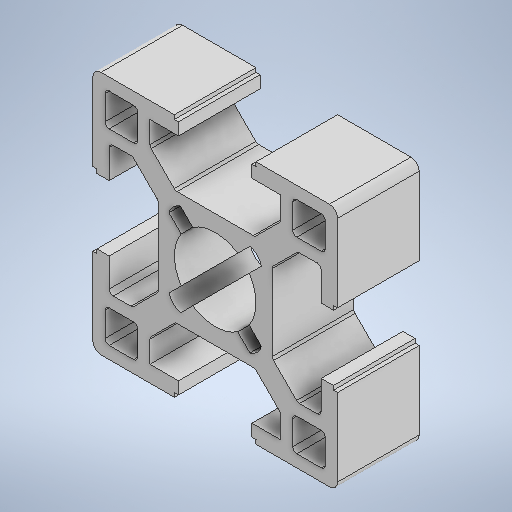
# Autodesk Inventor part: perfil_30x30_001
Saved by Autodesk Inventor 2026 (Build 300175000, 175)
## iProperties
Created: 2025-04-10
Part Number: perfil_30x30_001
Material: Generic
Document SubType Name: Modeling
Designer: Tony Dias
Density: 1 g/cm^3
Appearance: Default
Author: Tony Dias
Autodesk Inventor part; units mm, degrees
ref_plane "YZ Plane" through (0, 0, 0) normal (1, 0, 0) x (0, 1, 0)
ref_plane "XZ Plane" through (0, 0, 0) normal (0, 1, 0) x (-1, 0, 0)
ref_plane "XY Plane" through (0, 0, 0) normal (0, 0, 1) x (1, 0, 0)
sketch "Sketch1" plane through (0, 0, 0) normal (0, 0, 1) x (1, 0, 0)
  circle A0 centre (0, 0) radius 5 construction
  line L0 (-15, 15) -> (-4.5, 15) construction
  line L1 (-7, 7) -> (-7, 0) construction
  line L2 (-15, 15) -> (0, 0) construction
  line L3 (-7, 7) -> (0, 7) construction
  line L4 (-15, 15) -> (-15, 4) construction
  line L5 (-15, 4) -> (-13, 4) construction
  line L6 (-13.5, 13.5) -> (-9.5, 13.5)
  line L7 (-9.5, 13.5) -> (-9.5, 9.5)
  line L8 (-9.5, 9.5) -> (-13.5, 9.5)
  line L9 (-13.5, 9.5) -> (-13.5, 13.5)
  line L10 (-13.5, 13.5) -> (-9.5, 9.5) construction
  line L11 (-9.5, 13.5) -> (-13.5, 9.5) construction
  line L12 (-10.1213, 8) -> (-7, 4.8787)
  line L13 (-13, 8) -> (-10.1213, 8)
  line L14 (-13, 8) -> (-13, 4)
  line L15 (-7, 4.8787) -> (-7, 0)
  line L16 (-7, 0) -> (-5, 0)
  line L17 (-5.6712, 4.257) -> (-4.1712, 2.757)
  line L18 (-4.257, 5.6712) -> (-2.757, 4.1712)
  arc A1 (-4.257, 5.6712) -> (-5.6712, 4.257) centre (-3.7394, 3.7394) ccw
  arc A2 (0, 5) -> (-2.757, 4.1712) centre (0, 0) ccw
  arc A3 (-4.1712, 2.757) -> (-5, 0) centre (0, 0) ccw
  line L19 (-15, 4) -> (-14.5, 4) construction
  line L20 (-14.5, 4) -> (-14.5, 4.5)
  line L21 (-14.5, 4.5) -> (-15, 4.5)
  line L22 (-15, 4.5) -> (-15, 4) construction
  line L23 (-14.5, 4) -> (-13, 4)
  line L24 (-15, 15) -> (-15, 4.5)
  line L25 (-4.5, 15) -> (-4.5, 13) construction
  line L26 (-4.5, 13) -> (-8, 13)
  line L27 (-8, 13) -> (-8, 10.1213)
  line L28 (-8, 10.1213) -> (-4.8787, 7)
  line L29 (-4.8787, 7) -> (0, 7)
  line L30 (-4.5, 15) -> (-5, 15) construction
  line L31 (-5, 15) -> (-5, 14.5)
  line L32 (-5, 14.5) -> (-4.5, 14.5)
  line L33 (-4.5, 14.5) -> (-4.5, 15) construction
  line L34 (-4.5, 14.5) -> (-4.5, 13)
  line L35 (-15, 15) -> (-5, 15)
  line L36 (0, 7) -> (0, 5)
  point P0 (-11.5, 11.5)
  point P1 (-4.9212, 3.507)
  point P2 (-9.5, 11.5)
  dimension "d1" = 15
  dimension "d2" = 15
  dimension "d3" = 8
  dimension "d4" = 2
  dimension "d5" = 4
  dimension "d6" = 2
  dimension "d7" = 4
  dimension "d8" = 11.5
  dimension "d9" = 1.5
  dimension "d10" = 1.5
  dimension "d12" = 1.5
  dimension "d13" = 1
  dimension "d14" = 2
  dimension "d15" = 0.5
  dimension "d16" = 1.5
  constraints: 74 end point, 9 parallel, 9 point on circle, 8 equal length, 8 horizontal, 6 vertical, 5 collinear, 5 perpendicular, 4 centre point, 4 midpoint, 4 point on line, 3 concentric, 2 coincident, 2 vertical alignment, 1 horizontal alignment, 1 other
  measures "d1" horizontal distance of point (0, 0) L0.start
  measures "d2" horizontal distance of L0.start point (0, 0)
  measures "d3" distance from line of L0.start L1
  measures "d4" distance edge to line of A0 L1
  measures "d5" vertical distance of point (0, 0) L4.end
  measures "d6" distance of L4.end L5.end
  measures "d7" distance of L6.end L7.end
  measures "d8" horizontal distance of point (0, 0) point (-11.5, 11.5)
  measures "d9" distance between parallel lines of L2 L12
  measures "d10" distance between parallel lines of L8 L13
  measures "d12" horizontal distance of L17.start L17.end
  measures "d13" distance from line of L2 point (-4.921, 3.507)
  measures "d14" radius of A1
  measures "d15" distance of L20.end L21.end
  measures "d16" distance from line of point (-9.5, 11.5) L27
extrude "Extrusion1" add sketch "Sketch1" along normal mid plane 10
fillet "Fillet1" radius 1 1 edges at (-15, 15, 0)
fillet "Fillet2" radius 0.5 5 edges at (-8, 10.1213, 0) (-4.8787, 7, 0) (-7, 4.8787, 0) (-10.1213, 8, 0) (-13, 8, 0)
fillet "Fillet3" radius 0.5 4 edges at (-13.5, 13.5, 0) (-9.5, 13.5, 0) (-9.5, 9.5, 0) (-13.5, 9.5, 0)
mirror "Mirror1" about plane through (0, 0, 0) normal (1, 0, 0) of "Extrusion1", "Fillet1", "Fillet2", "Fillet3"
mirror "Mirror2" about plane through (0, 0, 0) normal (0, 1, 0) of "Extrusion1", "Fillet1", "Fillet2", "Fillet3", "Mirror1"
equation "\"d2\" = d1"
equation "\"d16\" = d10"
body "Solid1"
